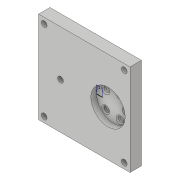
# Autodesk Inventor part: bottom part of capping system
Saved by Autodesk Inventor 2019 (Build 230136000, 136)
## iProperties
Created: 2019-10-12
Part Number: bottom part of capping system
Material: Generic
Document SubType Name: Modeling
Designer: Admin
Density: 1 g/cm^3
Appearance: Default
Author: Admin
Autodesk Inventor part; units mm, degrees
ref_plane "YZ Plane" through (0, 0, 0) normal (1, 0, 0) x (0, 1, 0)
ref_plane "XZ Plane" through (0, 0, 0) normal (0, 1, 0) x (-1, 0, 0)
ref_plane "XY Plane" through (0, 0, 0) normal (0, 0, 1) x (1, 0, 0)
sketch "Sketch1" plane through (0, 0, 0) normal (0, 0, 1) x (1, 0, 0)
  line L0 (0, 0) -> (160, 0)
  line L1 (160, 0) -> (160, 160)
  line L2 (160, 160) -> (0, 160)
  line L3 (0, 160) -> (0, 0)
  dimension "d0" = 160
  dimension "d1" = 160
  constraints: 8 end point, 2 parallel, 1 horizontal, 1 perpendicular
  measures "d0" distance of L2.end L1.end
  measures "d1" distance of L1.end L0.end
extrude "Extrusion1" add sketch "Sketch1" along normal blind 20
sketch "Sketch2" plane through (0, 0, 20) normal (0, 0, 1) x (1, 0, 0)
  line L0 (160, 160) -> (0, 160) projected
  line L1 (0, 160) -> (10, 160)
  line L2 (10, 160) -> (10, 10)
  line L3 (10, 10) -> (150, 10)
  line L4 (150, 10) -> (150, 150)
  line L5 (150, 150) -> (10, 150)
  circle A0 centre (10, 150) radius 5
  circle A1 centre (150, 150) radius 5
  circle A2 centre (10, 10) radius 5
  circle A3 centre (150, 10) radius 5
  line L6 (0, 0) -> (0, 80)
  line L7 (0, 160) -> (0, 0) projected
  line L8 (0, 80) -> (38.5, 80)
  circle A4 centre (38.5, 80) radius 5
  line L9 (0, 0) -> (160, 0) projected
  line L10 (160, 0) -> (160, 80)
  line L11 (160, 0) -> (160, 160) projected
  line L12 (160, 80) -> (160, 8)
  line L13 (160, 80) -> (121.5, 80)
  circle A5 centre (121.5, 80) radius 30
  dimension "d4" = 10
  dimension "d5" = 150
  dimension "d6" = 140
  dimension "d7" = 140
  dimension "d8" = 140
  dimension "d9" = 10
  dimension "d10" = 10
  dimension "d11" = 10
  dimension "d12" = 10
  dimension "d13" = 80
  dimension "d14" = 38.5
  dimension "d15" = 10
  dimension "d16" = 80
  dimension "d17" = 38.5
  dimension "d18" = 60
  constraints: 20 end point, 6 centre point, 6 coincident, 4 perpendicular, 3 point on line, 2 midpoint, 1 parallel
  measures "d4" distance of L0.end L1.end
  measures "d5" distance of L1.end L2.end
  measures "d6" distance of L2.end L3.end
  measures "d7" distance of L3.end L4.end
  measures "d8" distance of L4.end L5.end
  measures "d9" diameter of A0
  measures "d10" diameter of A1
  measures "d11" diameter of A2
  measures "d12" diameter of A3
  measures "d13" distance of L6.start L6.end
  measures "d14" distance of L6.end L8.end
  measures "d15" diameter of A4
  measures "d16" distance of L9.end L10.end
  measures "d17" distance of L10.end L13.end
  measures "d18" diameter of A5
extrude "Extrusion2" cut sketch "Sketch2" against normal through all contours A0 L5 L2 | L2 A0 | L5 A0 L2 | A1 L4 L5 | L5 L4 A1 | A3 L3 L4 | L4 L3 A3 | A2 L3 L2 | L2 L3 A2
sketch "Sketch3" plane through (0, 0, 20) normal (0, 0, 1) x (1, 0, 0)
  line L0 (0, 0) -> (160, 0) projected
  line L1 (0, 0) -> (0, 80)
  line L2 (0, 160) -> (0, 0) projected
  line L3 (0, 80) -> (38.5, 80)
  circle A0 centre (38.5, 80) radius 5
  line L4 (160, 0) -> (160, 11)
  dimension "d21" = 80
  dimension "d22" = 38.5
  dimension "d23" = 10
  constraints: 6 end point, 1 centre point, 1 coincident, 1 horizontal, 1 midpoint
  measures "d21" distance of L0.start L1.end
  measures "d22" distance of L1.end L3.end
  measures "d23" diameter of A0
extrude "Extrusion3" cut sketch "Sketch3" against normal blind 10
sketch "Sketch4" plane through (0, 0, 20) normal (0, 0, 1) x (1, 0, 0)
  line L0 (160, 0) -> (160, 160) projected
  line L1 (160, 0) -> (160, 80)
  line L2 (160, 80) -> (121.5, 80)
  circle A0 centre (121.5, 80) radius 30
  point P0 (0, 0)
  dimension "d26" = 80
  dimension "d27" = 38.5
  dimension "d28" = 60
  constraints: 4 end point, 1 centre point, 1 coincident, 1 midpoint, 1 perpendicular
  measures "d26" distance of L0.start L1.end
  measures "d27" distance of L1.end L2.end
  measures "d28" diameter of A0
extrude "Extrusion4" cut sketch "Sketch4" against normal blind 10
sketch "Sketch5" plane through (121.5, 80, 10) normal (0, 0, 1) x (1, 0, 0)
  line L0 (-30, 0) -> (-20, 0)
  line L1 (-20, 0) -> (-25, 0)
  point P0 (-121.5, -80)
  dimension "d31" = 10
  constraints: 4 end point, 1 horizontal, 1 midpoint
  measures "d31" distance of L0.start L0.end
sketch "Sketch6" plane through (121.5, 80, 10) normal (0, 0, 1) x (1, 0, 0)
  circle A0 centre (-14, -16) radius 5
  circle A1 centre (-14, 14) radius 5
  circle A2 centre (11, 19) radius 5
  circle A3 centre (22, -1) radius 5
  circle A4 centre (11, -19) radius 5
  point P0 (-121.5, -80)
  dimension "d32" = 10
  dimension "d33" = 10
  dimension "d34" = 10
  dimension "d35" = 10
  dimension "d36" = 10
  constraints: 5 centre point
  measures "d32" diameter of A0
  measures "d33" diameter of A1
  measures "d34" diameter of A2
  measures "d35" diameter of A3
  measures "d36" diameter of A4
extrude "Extrusion5" cut sketch "Sketch6" against normal blind 5
fillet "Fillet1" radius 2 5 edges at (102.5, 94, 10) (102.5, 64, 10) (127.5, 61, 10) (138.5, 79, 10) (127.5, 99, 10)
body "Solid1"
